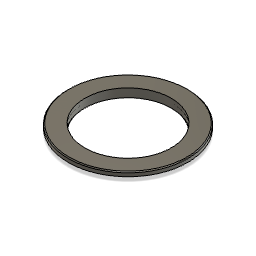
krouzek_svetlo_v1 (Autodesk Fusion 360 design; units mm, degrees)
Autodesk Fusion 360 part; units mm, degrees
sketch "Sketch1" plane through (0, 0, 0) normal (0, 1, 0) x (1, 0, 0)
  circle A0 centre (0, 0) radius 50.5
  circle A1 centre (0, 0) radius 70
  dimension "d1" = 101
  dimension "d2" = 140
  constraint coincident A0.centre A1.centre
  measures "d1" diameter of A0
  measures "d2" diameter of A1
extrude "Extrude1" add sketch "Sketch1" along normal blind 5
chamfer "Chamfer1" distance 1 angle 45 1 edges at (-65.2629, 5, 25.3131)
sketch "Sketch2" plane through (0, 0, 0) normal (0, -1, 0) x (1, 0, 0)
  circle A0 centre (0, 0) radius 50.5
  circle A1 centre (0, 0) radius 70
  circle A2 centre (0, 0) radius 50.5
  circle A3 centre (0, 0) radius 51.3
  dimension "d6" = 102.6
  constraint coincident A0.centre A1.centre
  constraint concentric A0 A3
  measures "d6" diameter of A3
extrude "Extrude2" add sketch "Sketch2" along normal blind 5 contours A3
equation "d6 = 101.000 mm + 0.8 * 2 mm"
